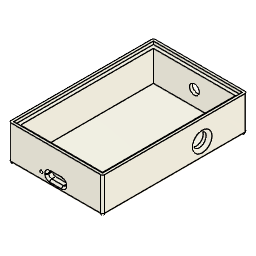
Luxmeter_case_V2.0 (Autodesk Fusion 360 design; units mm, degrees)
Autodesk Fusion 360 part; units mm, degrees
sketch "Sketch2" plane through (0, 0, 0) normal (0, 0, 1) x (1, 0, 0)
  line L0 (0, 74) -> (48, 74)
  line L1 (48, 74) -> (48, 0)
  line L2 (48, 0) -> (0, 0)
  line L3 (0, 0) -> (0, 74)
  dimension "d1" = 48
  dimension "d2" = 74
  constraint horizontal L0
  constraint vertical L1
  constraint horizontal L2
  constraint vertical L3
  measures "d1" distance of L0.start L0.end
  measures "d2" distance of L0.start L2.end
extrude "Extrude1" add sketch "Sketch2" along normal blind 18.6
sketch "Sketch5" plane through (0, 0, 18.6) normal (0, 0, 1) x (-1, 0, 0)
  line L0 (-3, -71) -> (-45, -71)
  line L1 (-45, -71) -> (-45, -3)
  line L2 (-45, -3) -> (-3, -3)
  line L3 (-3, -3) -> (-3, -71)
  dimension "d5" = 42
  dimension "d6" = 68
  constraint horizontal L0
  constraint vertical L1
  constraint horizontal L2
  constraint vertical L3
  measures "d5" distance of L0.start L0.end
  measures "d6" distance of L0.start L2.end
extrude "Extrude2" cut sketch "Sketch5" against normal blind 17
sketch "Sketch7" plane through (0, 0, 18.6) normal (0, 0, 1) x (-1, 0, 0)
  line L0 (-1.25, -72.75) -> (-46.75, -72.75)
  line L1 (-46.75, -72.75) -> (-46.75, -1.25)
  line L2 (-46.75, -1.25) -> (-1.25, -1.25)
  line L3 (-1.25, -1.25) -> (-1.25, -72.75)
  dimension "d9" = 45.5
  dimension "d10" = 71.5
  constraint horizontal L0
  constraint vertical L1
  constraint horizontal L2
  constraint vertical L3
  measures "d9" distance of L0.start L0.end
  measures "d10" distance of L0.start L2.end
extrude "Extrude3" cut sketch "Sketch7" against normal blind 1.5
sketch "Sketch8" plane through (0, 0, 0) normal (0, -1, 0) x (1, 0, 0)
  line L0 (20.9504, 6.5017) -> (27.0504, 6.5017)
  line L1 (28.5504, 5.0017) -> (28.5504, 4.7017)
  line L2 (27.0504, 3.2017) -> (20.9504, 3.2017)
  line L3 (19.4504, 4.7017) -> (19.4504, 5.0017)
  arc A0 (28.5504, 5.0017) -> (27.0504, 6.5017) centre (27.0504, 5.0017) ccw
  arc A1 (27.0504, 3.2017) -> (28.5504, 4.7017) centre (27.0504, 4.7017) ccw
  arc A2 (19.4504, 4.7017) -> (20.9504, 3.2017) centre (20.9504, 4.7017) ccw
  arc A3 (20.9504, 6.5017) -> (19.4504, 5.0017) centre (20.9504, 5.0017) ccw
  point P0 (19.4504, 6.5017)
  point P1 (28.5504, 6.5017)
  point P2 (19.4504, 3.2017)
  dimension "d13" = 9.1
  dimension "d14" = 3.3
  dimension "d15" = 1.5
  constraint horizontal L0
  constraint vertical L1
  constraint horizontal L2
  constraint vertical L3
  constraint coincident P1 L0
  constraint coincident P1 L1
  constraint tangent L0 A0
  constraint tangent L1 A0
  constraint tangent L1 A1
  constraint tangent L2 A1
  constraint equal A0 A1
  constraint coincident P2 L2
  constraint coincident P2 L3
  constraint tangent L2 A2
  constraint tangent L3 A2
  constraint equal A0 A2
  constraint coincident P0 L0
  constraint coincident P0 L3
  constraint tangent L0 A3
  constraint tangent L3 A3
  constraint equal A0 A3
  measures "d13" distance of P0 P1
  measures "d14" distance of P0 P2
  measures "d15" radius of A0
sketch "Sketch9" plane through (0, 0, 0) normal (0, -1, 0) x (1, 0, 0)
  circle A0 centre (16.6409, 4.6715) radius 0.75
  dimension "d16" = 1.5
  measures "d16" diameter of A0
extrude "Extrude4" cut sketch "Sketch9" against normal blind 3
extrude "Extrude5" cut sketch "Sketch8" against normal blind 3
sketch "Sketch10" plane through (48, 0, 0) normal (1, 0, 0) x (0, 1, 0)
  circle A0 centre (51, 8.3) radius 3.5
  dimension "d21" = 7
  measures "d21" diameter of A0
extrude "Extrude6" cut sketch "Sketch10" against normal blind 3
sketch "Sketch11" plane through (0, 71, 0) normal (0, -1, 0) x (1, 0, 0)
  circle A0 centre (24, 9.35) radius 2.5
  dimension "d24" = 5
  measures "d24" diameter of A0
extrude "Extrude7" cut sketch "Sketch11" against normal blind 3
fillet "Fillet1" radius 1.5 1 edges at (21.6692, 74, 8.446)
fillet "Fillet2" radius 1.5 1 edges at (48, 47.7369, 9.5657)
fillet "Fillet3" radius 1 8 edges at (28.5504, 0, 4.8517) (28.1111, 0, 3.6411) (24.0004, 0, 3.2017) (19.8898, 0, 3.6411) (19.4504, 0, 4.8517) (19.8898, 0, 6.0624) (24.0004, 0, 6.5017) (28.1111, 0, 6.0624)
fillet "Fillet4" radius 1 4 edges at (48, 0, 9.3) (0, 0, 9.3) (0, 74, 9.3) (48, 74, 9.3)
fillet "Fillet5" radius 1.5 8 edges at (47.7071, 73.7071, 0) (48, 37, 0) (47.7071, 0.2929, 0) (24, 0, 0) (0.2929, 0.2929, 0) (0, 37, 0) (0.2929, 73.7071, 0) (24, 74, 0)
sketch "Sketch12" plane through (0, 0, 0) normal (0, 0, -1) x (1, 0, 0)
  line L0 (26, -65) -> (1.8029, -65.0911) construction
  line L1 (1.8029, -65.0911) -> (1.8302, -72.3569) construction
  line L2 (1.8302, -72.3569) -> (26.0274, -72.2658) construction
  line L3 (26.0274, -72.2658) -> (26, -65) construction
  dimension "d37" = 5
  dimension "d38" = 0
  text T0 "V 2.0" font "Arial Black" height 5 align centre bottom in box 24.1973 x 7.2659 at (26, -65) x (-0.999993, -0.003764) y (0.003764, -0.999993) spacing 1 kerned
extrude "Extrude8" cut sketch "Sketch12" against normal blind 1 text T0
equation "d38 = 'V 2.0'"
